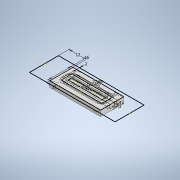
# Autodesk Inventor part: Capping_Insert
Saved by Autodesk Inventor 2022 (Build 260153000, 153)
## iProperties
Created: 2024-04-10
Part Number: Capping_Insert
Material: Generic
Document SubType Name: Modeling
Designer: Gotham City
Density: 1 g/cm^3
Appearance: Default
Author: Gotham City
Autodesk Inventor part; units mm, degrees
ref_plane "YZ Plane" through (0, 0, 0) normal (1, 0, 0) x (0, 1, 0)
ref_plane "XZ Plane" through (0, 0, 0) normal (0, 1, 0) x (-1, 0, 0)
ref_plane "XY Plane" through (0, 0, 0) normal (0, 0, 1) x (1, 0, 0)
sketch "Sketch1" plane through (0, 0, 0) normal (0, 1, 0) x (-1, 0, 0)
  line L0 (13.925, -3.65) -> (-13.925, -3.65)
  line L1 (-13.925, -3.65) -> (-13.925, 3.65)
  line L2 (-13.925, 3.65) -> (13.925, 3.65)
  line L3 (13.925, 3.65) -> (13.925, -3.65)
  line L4 (13.925, -3.65) -> (-13.925, 3.65) construction
  line L5 (-13.925, -3.65) -> (13.925, 3.65) construction
  line L6 (11.725, -1.25) -> (-11.725, -1.25)
  line L7 (-11.725, -1.25) -> (-11.725, 1.25)
  line L8 (-11.725, 1.25) -> (11.725, 1.25)
  line L9 (11.725, 1.25) -> (11.725, -1.25)
  line L10 (11.725, -1.25) -> (-11.725, 1.25) construction
  line L11 (-11.725, -1.25) -> (11.725, 1.25) construction
  line L12 (11.725, -1.25) -> (11.725, -3.65) construction
  line L13 (11.725, 1.25) -> (11.725, 3.65) construction
  line L14 (11.725, -1.25) -> (13.925, -1.25) construction
  line L15 (-11.725, -1.25) -> (-13.925, -1.25) construction
  point P0 (0, 0)
  point P1 (0, 0)
  point P2 (0, 0)
  point P3 (0, 0)
  dimension "d0" = 27.85
  dimension "d1" = 7.3
  dimension "d2" = 2.4
  dimension "d3" = 2.4
  dimension "d4" = 2.5
  dimension "d5" = 2.2
  dimension "d6" = 23.45
  constraints: 32 end point, 6 point on line, 5 midpoint, 4 parallel, 4 perpendicular, 2 collinear, 2 horizontal, 1 coincident
  measures "d0" distance of L0.start L0.end
  measures "d1" distance of L0.end L1.end
  measures "d2" distance between parallel lines of L0 L6
  measures "d3" distance between parallel lines of L2 L8
  measures "d4" distance of L6.end L7.end
  measures "d5" distance of L6.end L15.end
  measures "d6" distance of L6.start L6.end
sketch "Sketch2" plane through (0, 0, 0) normal (0, 1, 0) x (-1, 0, 0)
  line L0 (17.5, 8) -> (-17.5, 8)
  line L1 (-17.5, 8) -> (-17.5, -8)
  line L2 (-17.5, -8) -> (17.5, -8)
  line L3 (17.5, -8) -> (17.5, 8)
  line L4 (17.5, 8) -> (-17.5, -8) construction
  point P0 (0, 0)
  point P1 (0, 0)
  dimension "d7" = 35
  dimension "d8" = 16
  constraints: 10 end point, 2 parallel, 1 coincident, 1 horizontal, 1 midpoint, 1 perpendicular
  measures "d7" distance of L0.start L0.end
  measures "d8" distance of L2.end L0.start
extrude "Extrusion1" add sketch "Sketch2" against normal blind 4
sketch "Sketch5" plane through (0, 0, 0) normal (0, 1, 0) x (1, 0, 0)
  line L0 (-12.925, -2.45) -> (12.925, -2.45)
  line L1 (12.925, -2.45) -> (12.925, 2.45)
  line L2 (12.925, 2.45) -> (-12.925, 2.45)
  line L3 (-12.925, 2.45) -> (-12.925, -2.45)
  line L4 (-12.925, -2.45) -> (12.925, 2.45) construction
  line L5 (11.725, -1.25) -> (-11.725, -1.25) construction
  line L6 (-11.725, 1.25) -> (11.725, 1.25) construction
  line L7 (24.5, 0) -> (-24.5, 0) construction
  line L8 (0, 11.2) -> (0, -11.2) construction
  point P0 (0, 0)
  point P1 (0, 0)
  dimension "d11" = 1.2
  dimension "d12" = 1.2
  constraints: 10 end point, 2 parallel, 1 coincident, 1 horizontal, 1 midpoint, 1 perpendicular, 2 other
  measures "d11" distance between parallel lines of L5 L0
  measures "d12" distance from line of L3 L5.end
extrude "Extrusion2" cut sketch "Sketch5" against normal blind 2
fillet "Fillet1" radius 1.2 4 edges at (12.925, -1, 2.45) (-12.925, -1, 2.45) (-12.925, -1, -2.45) (12.925, -1, -2.45)
sketch "Sketch6" plane through (0, 0, 0) normal (0, 1, 0) x (1, 0, 0)
  arc A0 (12.925, 1.25) -> (11.725, 2.45) centre (11.725, 1.25) ccw projected
  line L0 (-11.725, 2.45) -> (11.725, 2.45) projected
  arc A1 (-11.725, 2.45) -> (-12.925, 1.25) centre (-11.725, 1.25) ccw projected
  line L1 (-12.925, -1.25) -> (-12.925, 1.25) projected
  arc A2 (-12.925, -1.25) -> (-11.725, -2.45) centre (-11.725, -1.25) ccw projected
  line L2 (11.725, -2.45) -> (-11.725, -2.45) projected
  arc A3 (11.725, -2.45) -> (12.925, -1.25) centre (11.725, -1.25) ccw projected
  line L3 (12.925, 1.25) -> (12.925, -1.25) projected
  arc A4 (14.425, 1.25) -> (11.725, 3.95) centre (11.725, 1.25) ccw
  line L4 (14.425, 1.25) -> (14.425, -1.25)
  arc A5 (11.725, -3.95) -> (14.425, -1.25) centre (11.725, -1.25) ccw
  line L5 (11.725, -3.95) -> (-11.725, -3.95)
  arc A6 (-14.425, -1.25) -> (-11.725, -3.95) centre (-11.725, -1.25) ccw
  line L6 (-14.425, -1.25) -> (-14.425, 1.25)
  arc A7 (-11.725, 3.95) -> (-14.425, 1.25) centre (-11.725, 1.25) ccw
  line L7 (-11.725, 3.95) -> (11.725, 3.95)
  line L8 (-15.625, 1.25) -> (-15.625, -1.25)
  arc A8 (-15.625, -1.25) -> (-11.725, -5.15) centre (-11.725, -1.25) ccw
  line L9 (-11.725, -5.15) -> (11.725, -5.15)
  arc A9 (11.725, -5.15) -> (15.625, -1.25) centre (11.725, -1.25) ccw
  line L10 (15.625, -1.25) -> (15.625, 1.25)
  arc A10 (15.625, 1.25) -> (11.725, 5.15) centre (11.725, 1.25) ccw
  line L11 (11.725, 5.15) -> (-11.725, 5.15)
  arc A11 (-11.725, 5.15) -> (-15.625, 1.25) centre (-11.725, 1.25) ccw
  point P0 (0, 0)
  dimension "d16" = 1.5
  dimension "d17" = 1.2
  constraints: 16 end point, 16 point on circle, 8 centre point, 14 other
  measures "d16" distance between parallel lines of L7 L0
  measures "d17" radial gap between concentric circles of A7 A11
extrude "Extrusion3" cut sketch "Sketch6" against normal blind 0.6 contours A11 L11 A10 L10 A9 L9 A8 L8
sketch "Sketch7" plane through (0, 0, 0) normal (0, 1, 0) x (1, 0, 0)
  line L0 (-29.5, -10) -> (29.5, -10)
  line L1 (29.5, -10) -> (29.5, 10)
  line L2 (29.5, 10) -> (-29.5, 10)
  line L3 (-29.5, 10) -> (-29.5, -10)
  line L4 (-41.3, 0) -> (41.3, 0) construction
  line L5 (0, 14) -> (0, -14) construction
  line L6 (-17.5, 8) -> (-17.5, -8) construction
  line L7 (17.5, 8) -> (-17.5, 8) construction
  point P0 (0, 0)
  dimension "d20" = 12
  dimension "d21" = 2
  constraints: 8 end point, 2 parallel, 1 horizontal, 1 perpendicular, 2 other
  measures "d20" distance between parallel lines of L3 L6
  measures "d21" distance between parallel lines of L2 L7
equation "\"d12\" = d11"
body "Solid1"
